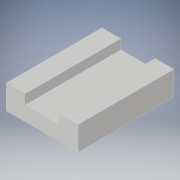
# Autodesk Inventor part: RS-FixedFiber
Saved by Autodesk Inventor 2019 (Build 230136000, 136)
## iProperties
Created: 2019-06-18
Part Number: RS-FixedFiber
Material: Generic
Document SubType Name: Modeling
Designer: aorfi
Density: 1 g/cm^3
Appearance: Default
Author: aorfi
Autodesk Inventor part; units mm, degrees
ref_plane "YZ Plane" through (0, 0, 0) normal (1, 0, 0) x (0, 1, 0)
ref_plane "XZ Plane" through (0, 0, 0) normal (0, 1, 0) x (-1, 0, 0)
ref_plane "XY Plane" through (0, 0, 0) normal (0, 0, 1) x (1, 0, 0)
sketch "Sketch1" plane through (0, 0, 0) normal (0, 1, 0) x (-1, 0, 0)
  line L0 (-7.5, 10) -> (7.5, 10)
  line L1 (7.5, 10) -> (7.5, -10)
  line L2 (7.5, -10) -> (-7.5, -10)
  line L3 (-7.5, -10) -> (-7.5, 10)
  line L4 (-7.5, 10) -> (7.5, -10) construction
  line L5 (7.5, 10) -> (-7.5, -10) construction
  point P0 (0, 0)
  dimension "d0" = 20
  dimension "d1" = 15
  constraints: 12 end point, 2 midpoint, 2 parallel, 1 horizontal, 1 perpendicular
  measures "d0" distance of L0.end L1.end
  measures "d1" distance of L1.end L2.end
extrude "Extrusion1" add sketch "Sketch1" along normal mid plane 3
sketch "Sketch2" plane through (0, 1.5, 0) normal (0, 1, 0) x (1, 0, 0)
  line L0 (-7.5, -10) -> (7.5, -10) projected
  line L1 (7.5, -10) -> (7.5, 10) projected
  line L2 (7.5, 10) -> (-7.5, 10) projected
  line L3 (-7.5, 10) -> (-7.5, -10) projected
  line L4 (-3.565, -10) -> (3.565, -10)
  line L5 (3.565, -10) -> (3.565, 10)
  line L6 (3.565, 10) -> (-3.565, 10)
  line L7 (-3.565, 10) -> (-3.565, -10)
  point P0 (0, 0)
  point P1 (0, 10)
  dimension "d5" = 7.13
  constraints: 8 end point, 2 parallel, 2 point on line, 1 horizontal, 1 midpoint, 1 perpendicular, 1 vertical alignment
  measures "d5" distance between parallel lines of L5 L7
extrude "Extrusion2" add sketch "Sketch2" along normal blind 2 contours L3 L2 L7 L0 | L5 L2 L1 L0
body "Solid1"
